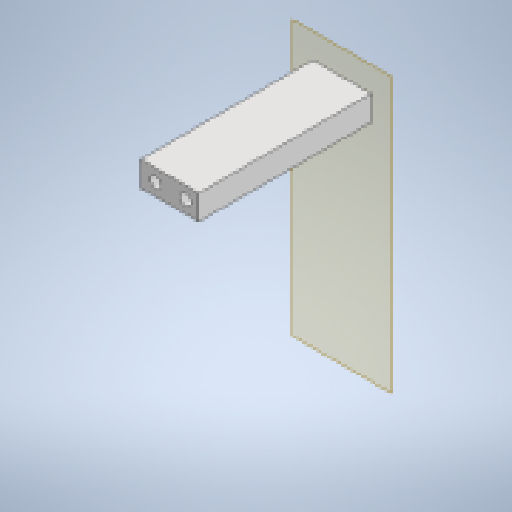
# Autodesk Inventor part: _fist_ver2_
Saved by Autodesk Inventor 2024.3 (Build 283343000, 343)
## iProperties
Created: 2024-09-07
Part Number: _fist_ver2_
Material: 일반
Document SubType Name: Modeling
Designer: gretc
Density: 1 g/cm^3
Appearance: 기본값
Author: gretc
Autodesk Inventor part; units mm, degrees
ref_plane "YZ Plane" through (0, 0, 0) normal (1, 0, 0) x (0, 1, 0)
ref_plane "XZ Plane" through (0, 0, 0) normal (0, 1, 0) x (-1, 0, 0)
ref_plane "XY Plane" through (0, 0, 0) normal (0, 0, 1) x (1, 0, 0)
ref_plane "작업 평면1" through (0, 0, 0) normal (0, 0, 1) x (1, 0, 0)
sketch "스케치1" plane through (0, 0, 0) normal (0, 0, 1) x (1, 0, 0)
  line L0 (-10.4523, 80.0529) -> (11.1476, 79.9778) projected
  line L1 (-10.7999, -19.9465) -> (-10.4523, 80.0529) projected
  arc A0 (-10.7999, -19.9465) -> (-4.0349, -30.002) centre (0, -19.984) ccw projected
  line L2 (-4, -19.9701) -> (-4.0349, -30.002) projected
  arc A1 (4, -19.9979) -> (-4, -19.9701) centre (0, -19.984) ccw projected
  line L3 (3.9651, -30.0298) -> (4, -19.9979) projected
  arc A2 (3.9651, -30.0298) -> (10.7999, -20.0216) centre (0, -19.984) ccw projected
  line L4 (11.1476, 79.9778) -> (10.7999, -20.0216) projected
  circle A3 centre (-8, -19.9562) radius 1.05 projected
  circle A4 centre (-5.6372, -14.3075) radius 1.05 projected
  circle A5 centre (0.0278, -11.9841) radius 1.05 projected
  circle A6 centre (5.6765, -14.3469) radius 1.05 projected
  circle A7 centre (-3.2732, 74.0279) radius 1.35 projected
  circle A8 centre (3.9268, 74.0029) radius 1.35 projected
  circle A9 centre (5.6372, -25.6605) radius 1.05 projected
  circle A10 centre (-5.6765, -25.6212) radius 1.05 projected
  circle A11 centre (8, -20.0118) radius 1.05 projected
  line L5 (3.9268, 74.0029) -> (3.9268, 77.0029)
  line L6 (3.9268, 74.0029) -> (6.9268, 74.0029) construction
  line L7 (3.9268, 74.0029) -> (3.9268, 71.0029)
  line L8 (3.9268, 74.0029) -> (6.9268, 74.0029) construction
  line L9 (3.9268, 74.0029) -> (0, 74.0029)
  line L10 (-7, 77.0029) -> (7, 77.0029)
  line L11 (7, 77.0029) -> (7, 71.0029)
  line L12 (7, 71.0029) -> (-7, 71.0029)
  line L13 (-7, 71.0029) -> (-7, 77.0029)
  line L14 (-7, 77.0029) -> (7, 71.0029) construction
  line L15 (7, 77.0029) -> (-7, 71.0029) construction
  point P0 (0, 0)
  dimension "d0" = 3
  dimension "d1" = 90
  dimension "d2" = 3
  dimension "d3" = 90
  dimension "d4" = 14
  constraints: 22 end point, 3 horizontal, 3 perpendicular, 2 midpoint, 2 parallel, 2 vertical
  measures "d0" distance of L5.start L5.end
  measures "d1" angle of L6 L5
  measures "d2" distance of L5.start L7.end
  measures "d3" angle of L7 L8
  measures "d4" distance of L10.start L10.end
ref_plane "작업 평면2" through (-10.8348, -30.0535, 41.45) normal (0, 0, -1) x (0.0034767, 0.999994, 0)
extrude "돌출1" add sketch "스케치1" along normal up to surface (41.45 mm away) contours A8 L5 L10 L11 L12 L7 | A8 L7 L12 L13 L10 L5
